Autodesk Inventor part; units mm, degrees
(part 4 of 4)
sketch "スケッチ30" plane through (0, 0, -5) normal (0, 0, -1) x (-1, 0, 0)
  arc A0 (-103.5253, -51.4545) -> (-102.2194, -50.4706) centre (-111.885, -39) ccw projected
  arc A1 (-103.5253, -51.4545) -> (-102.968, -53.2848) centre (-102.968, -52.2848) ccw projected
  line L0 (-102.968, -53.2848) -> (-61.8586, -53.2848) projected
  arc A2 (-61.8586, -53.2848) -> (-61.1613, -51.5681) centre (-61.8586, -52.2848) ccw projected
  line L1 (-61.1613, -51.5681) -> (-80.173, -33.0718) projected
  arc A3 (-80.173, -33.0718) -> (-81.5147, -33.0239) centre (-80.8703, -33.7886) ccw projected
  line L2 (-81.5147, -33.0239) -> (-102.2194, -50.4706) projected
  arc A4 (-99.1877, -14.5726) -> (-100.885, -15.2893) centre (-99.885, -15.2893) ccw projected
  line L3 (-100.885, -15.2893) -> (-100.885, -31.7889) projected
  arc A5 (-100.885, -31.7889) -> (-100.7422, -32.304) centre (-99.885, -31.7889) ccw projected
  arc A6 (-98.9442, -40.2383) -> (-100.7422, -32.304) centre (-111.885, -39) ccw projected
  arc A7 (-98.9442, -40.2383) -> (-97.3043, -41.0982) centre (-97.9487, -40.3335) ccw projected
  line L4 (-97.3043, -41.0982) -> (-84.5476, -30.3488) projected
  arc A8 (-84.5476, -30.3488) -> (-84.4946, -28.8673) centre (-85.1919, -29.5841) ccw projected
  line L5 (-84.4946, -28.8673) -> (-99.1877, -14.5726) projected
  arc A9 (-82.0469, -27.0631) -> (-80.7052, -27.1111) centre (-81.3496, -26.3464) ccw projected
  line L6 (-80.7052, -27.1111) -> (-61.3064, -10.7647) projected
  arc A10 (-61.3064, -10.7647) -> (-61.9507, -9) centre (-61.9507, -10) ccw projected
  line L7 (-61.9507, -9) -> (-62.4443, -9) projected
  arc A11 (-62.4443, -9) -> (-63.0443, -9.2) centre (-62.4443, -10) ccw projected
  arc A12 (-69.1163, -7.5865) -> (-63.0443, -9.2) centre (-65.4443, -6) ccw projected
  arc A13 (-69.1163, -7.5865) -> (-70.1163, -6.9865) centre (-70.0342, -7.9832) ccw projected
  arc A14 (-72.8443, -6.2) -> (-70.1163, -6.9865) centre (-70.4443, -3) ccw projected
  arc A15 (-72.8443, -6.2) -> (-73.4443, -6) centre (-73.4443, -7) ccw projected
  line L8 (-73.4443, -6) -> (-80.8897, -6) projected
  arc A16 (-80.8897, -6) -> (-81.4897, -6.2) centre (-80.8897, -7) ccw projected
  arc A17 (-84.2178, -6.9865) -> (-81.4897, -6.2) centre (-83.8897, -3) ccw projected
  arc A18 (-84.2178, -6.9865) -> (-85.2178, -7.5865) centre (-84.2998, -7.9832) ccw projected
  arc A19 (-91.2897, -9.2) -> (-85.2178, -7.5865) centre (-88.8897, -6) ccw projected
  arc A20 (-91.2897, -9.2) -> (-91.8897, -9) centre (-91.8897, -10) ccw projected
  line L9 (-91.8897, -9) -> (-92.8897, -9) projected
  arc A21 (-92.8897, -9) -> (-93.4897, -9.2) centre (-92.8897, -10) ccw projected
  arc A22 (-97.0553, -9.8264) -> (-93.4897, -9.2) centre (-95.8897, -6) ccw projected
  arc A23 (-97.0553, -9.8264) -> (-98.044, -11.4998) centre (-97.3467, -10.783) ccw projected
  line L10 (-98.044, -11.4998) -> (-82.0469, -27.0631) projected
  circle A24 centre (-90.0199, -69.8335) radius 1.5 projected
  circle A25 centre (-49.9722, -10.5) radius 1.5 projected
  arc A26 (-109.4606, -24.6009) -> (-107.885, -23.7831) centre (-108.885, -23.7831) ccw projected
  line L11 (-109.4606, -24.6009) -> (-113.2999, -21.8986) projected
  arc A27 (-113.5421, -20.5053) -> (-113.2999, -21.8986) centre (-112.7243, -21.0809) ccw projected
  line L12 (-113.5421, -20.5053) -> (-109.7028, -15.0506) projected
  arc A28 (-107.885, -15.6261) -> (-109.7028, -15.0506) centre (-108.885, -15.6261) ccw projected
  line L13 (-107.885, -15.6261) -> (-107.885, -23.7831) projected
  arc A29 (-118.0918, -32.7971) -> (-116.8906, -32.7594) centre (-117.5163, -31.9794) ccw projected
  line L14 (-118.0918, -32.7971) -> (-120.017, -31.4421) projected
  arc A30 (-120.2592, -30.0488) -> (-120.017, -31.4421) centre (-119.4414, -30.6244) ccw projected
  line L15 (-120.2592, -30.0488) -> (-116.4199, -24.5941) projected
  arc A31 (-115.0266, -24.3519) -> (-116.4199, -24.5941) centre (-115.6022, -25.1696) ccw projected
  line L16 (-115.0266, -24.3519) -> (-108.3095, -29.0797) projected
  arc A32 (-107.885, -29.8974) -> (-108.3095, -29.0797) centre (-108.885, -29.8974) ccw projected
  line L17 (-107.885, -29.8974) -> (-107.885, -30.5147) projected
  arc A33 (-109.2184, -31.4575) -> (-107.885, -30.5147) centre (-108.885, -30.5147) ccw projected
  arc A34 (-109.2184, -31.4575) -> (-116.8906, -32.7594) centre (-111.885, -39) ccw projected
  arc A35 (-121.5083, -34.0611) -> (-123.011, -34.5042) centre (-122.0839, -34.8788) ccw projected
  line L18 (-121.5083, -34.0611) -> (-119.8185, -35.2504) projected
  arc A36 (-119.4487, -36.3939) -> (-119.8185, -35.2504) centre (-120.3941, -36.0681) ccw projected
  arc A37 (-119.4487, -36.3939) -> (-119.4653, -41.5573) centre (-111.885, -39) ccw projected
  arc A38 (-120.4273, -42.8769) -> (-119.4653, -41.5573) centre (-120.4128, -41.877) ccw projected
  line L19 (-120.4273, -42.8769) -> (-123.2447, -42.8361) projected
  arc A39 (-124.2252, -41.735) -> (-123.2447, -42.8361) centre (-123.2303, -41.8362) ccw projected
  line L20 (-124.2252, -41.735) -> (-123.8235, -37.7857) projected
  arc A40 (-123.011, -34.5042) -> (-123.8235, -37.7857) centre (-111.885, -39) ccw projected
  arc A41 (-59.9987, -48.5136) -> (-58.3014, -47.7969) centre (-59.3014, -47.7969) ccw projected
  line L21 (-58.3014, -47.7969) -> (-58.3014, -15.6137) projected
  arc A42 (-58.3014, -15.6137) -> (-59.9457, -14.8489) centre (-59.3014, -15.6137) ccw projected
  line L22 (-59.9457, -14.8489) -> (-77.6723, -29.7862) projected
  arc A43 (-77.6723, -29.7862) -> (-77.7253, -31.2676) centre (-77.0279, -30.5509) ccw projected
  line L23 (-77.7253, -31.2676) -> (-59.9987, -48.5136) projected
  arc A44 (-65.1718, -84.4734) -> (-63.9261, -84.9061) centre (-64.3023, -83.9795) ccw projected
  line L24 (-63.9261, -84.9061) -> (-58.9251, -82.8752) projected
  arc A45 (-58.9251, -82.8752) -> (-58.3014, -81.9487) centre (-59.3014, -81.9487) ccw projected
  line L25 (-58.3014, -81.9487) -> (-58.3014, -57.2848) projected
  arc A46 (-58.3014, -57.2848) -> (-59.3014, -56.2848) centre (-59.3014, -57.2848) ccw projected
  line L26 (-59.3014, -56.2848) -> (-101.5991, -56.2848) projected
  arc A47 (-101.5991, -56.2848) -> (-102.1316, -58.1313) centre (-101.5991, -57.2848) ccw projected
  line L27 (-102.1316, -58.1313) -> (-90.9084, -65.1915) projected
  arc A48 (-90.9084, -65.1915) -> (-90.3112, -65.343) centre (-90.376, -64.3451) ccw projected
  arc A49 (-85.8458, -68.1521) -> (-90.3112, -65.343) centre (-90.0199, -69.8335) ccw projected
  arc A50 (-85.8458, -68.1521) -> (-85.4507, -68.6249) centre (-84.9182, -67.7784) ccw projected
  line L28 (-85.4507, -68.6249) -> (-72.5868, -76.7173) projected
  arc A51 (-65.1718, -84.4734) -> (-72.5868, -76.7173) centre (-84.3014, -95.339) ccw projected
  arc A52 (-62.421, -88.6121) -> (-63.0125, -89.7908) centre (-62.0448, -89.5386) ccw projected
  arc A53 (-62.7437, -90.9495) -> (-63.0125, -89.7908) centre (-84.3014, -95.339) ccw projected
  arc A54 (-62.7437, -90.9495) -> (-61.7638, -91.75) centre (-61.7638, -90.75) ccw projected
  line L29 (-61.7638, -91.75) -> (-55.2884, -91.75) projected
  arc A55 (-55.2884, -91.75) -> (-54.9084, -91.675) centre (-55.2884, -90.75) ccw projected
  line L30 (-54.9084, -91.675) -> (-53.6916, -91.1751) projected
  arc A56 (-53.6916, -91.1751) -> (-53.1201, -89.9424) centre (-54.0715, -90.2501) ccw projected
  arc A57 (-53.3763, -88.5912) -> (-53.1201, -89.9424) centre (-47.8869, -88.25) ccw projected
  arc A58 (-53.3763, -88.5912) -> (-54.1956, -87.6694) centre (-54.3744, -88.6533) ccw projected
  arc A59 (-56.3726, -86.6955) -> (-54.1956, -87.6694) centre (-53.3014, -82.75) ccw projected
  arc A60 (-56.3726, -86.6955) -> (-57.3632, -86.5581) centre (-56.9869, -87.4846) ccw projected
  line L31 (-57.3632, -86.5581) -> (-62.421, -88.6121) projected
  circle A61 centre (-47.8869, -88.25) radius 1.5 projected
  line L32 (-127.6513, -45.7727) -> (-119.127, -45.896) projected
  arc A62 (-119.127, -45.896) -> (-104.885, -31.8586) centre (-111.885, -39) ccw projected
  line L33 (-104.885, -31.8586) -> (-104.885, -3) projected
  line L34 (-104.885, -3) -> (-101.8897, -3) projected
  arc A63 (-101.8897, -3) -> (-99.8897, -3) centre (-100.8897, -3) ccw projected
  line L35 (-99.8897, -3) -> (-96.8897, -3) projected
  line L36 (-96.8897, -3) -> (-96.8897, -6) projected
  arc A64 (-96.8897, -6) -> (-94.8897, -6) centre (-95.8897, -6) ccw projected
  line L37 (-94.8897, -6) -> (-89.8897, -6) projected
  arc A65 (-89.8897, -6) -> (-87.8897, -6) centre (-88.8897, -6) ccw projected
  line L38 (-87.8897, -6) -> (-87.8897, -3) projected
  line L39 (-87.8897, -3) -> (-84.8897, -3) projected
  arc A66 (-84.8897, -3) -> (-82.8897, -3) centre (-83.8897, -3) ccw projected
  line L40 (-82.8897, -3) -> (-71.4443, -3) projected
  arc A67 (-71.4443, -3) -> (-69.4443, -3) centre (-70.4443, -3) ccw projected
  line L41 (-69.4443, -3) -> (-66.4443, -3) projected
  line L42 (-66.4443, -3) -> (-66.4443, -6) projected
  arc A68 (-66.4443, -6) -> (-64.4443, -6) centre (-65.4443, -6) ccw projected
  line L43 (-64.4443, -6) -> (-59.4443, -6) projected
  arc A69 (-59.4443, -6) -> (-57.4443, -6) centre (-58.4443, -6) ccw projected
  line L44 (-57.4443, -6) -> (-57.4443, -3) projected
  line L45 (-57.4443, -3) -> (-54.4443, -3) projected
  arc A70 (-54.4443, -3) -> (-52.4443, -3) centre (-53.4443, -3) ccw projected
  line L46 (-52.4443, -3) -> (-49.4443, -3) projected
  line L47 (-49.4443, -3) -> (-49.4443, -5.2165) projected
  arc A71 (-49.4443, -5.2165) -> (-48.7221, -6.1771) centre (-48.4443, -5.2165) ccw projected
  arc A72 (-52.6961, -14.082) -> (-48.7221, -6.1771) centre (-49.9722, -10.5) ccw projected
  arc A73 (-52.6961, -14.082) -> (-54.3014, -14.878) centre (-53.3014, -14.878) ccw projected
  line L48 (-54.3014, -14.878) -> (-54.3014, -82.75) projected
  arc A74 (-54.3014, -82.75) -> (-53.3014, -83.75) centre (-53.3014, -82.75) ccw projected
  line L49 (-53.3014, -83.75) -> (-47.885, -83.75) projected
  arc A75 (-46.177, -92.4125) -> (-47.885, -83.75) centre (-47.8869, -88.25) ccw projected
  line L50 (-46.177, -92.4125) -> (-54.3014, -95.75) projected
  line L51 (-54.3014, -95.75) -> (-66.3014, -95.75) projected
  line L52 (-66.3014, -95.75) -> (-66.3014, -95.339) projected
  arc A76 (-66.3014, -95.339) -> (-74.7167, -80.1031) centre (-84.3014, -95.339) ccw projected
  line L53 (-74.7167, -80.1031) -> (-85.8413, -73.1048) projected
  arc A77 (-85.8413, -73.1048) -> (-87.0367, -73.2026) centre (-86.3737, -73.9513) ccw projected
  arc A78 (-94.3483, -68.603) -> (-87.0367, -73.2026) centre (-90.0199, -69.8335) ccw projected
  arc A79 (-94.3483, -68.603) -> (-94.7777, -67.4831) centre (-95.3102, -68.3295) ccw projected
  line L54 (-94.7777, -67.4831) -> (-119.8722, -51.6966) projected
  arc A80 (-121.0577, -50.8686) -> (-119.8722, -51.6966) centre (-111.885, -39) ccw projected
  line L55 (-121.0577, -50.8686) -> (-127.6513, -45.7727) projected
  arc A81 (-52.6961, -14.082) -> (-54.3014, -14.878) centre (-53.3014, -14.878) ccw projected
  circle A82 centre (-49.9722, -10.5) radius 4.5
  line L56 (-54.3014, -14.878) -> (-54.3014, -9.2717)
  line L57 (-49.4443, -5.2165) -> (-49.4443, -3) projected
  line L58 (-49.4443, -5.2165) -> (-49.4443, -6.0311)
  point P0 (0, 0)
  constraints: 4 end point, 3 point on circle, 2 collinear, 1 centre point, 1 coincident
extrude "押し出し30" cut sketch "スケッチ30" against normal blind 2 contours L56 A82 A73 | A82 L56 A72 | A82 L58 A71
fillet "フィレット10" radius 1 1 edges at (54.3014, -9.2717, -4)
sketch "スケッチ31" plane through (0, 0, -5) normal (0, 0, -1) x (-1, 0, 0)
  arc A0 (-103.5253, -51.4545) -> (-102.2194, -50.4706) centre (-111.885, -39) ccw projected
  arc A1 (-103.5253, -51.4545) -> (-102.968, -53.2848) centre (-102.968, -52.2848) ccw projected
  line L0 (-102.968, -53.2848) -> (-61.8586, -53.2848) projected
  arc A2 (-61.8586, -53.2848) -> (-61.1613, -51.5681) centre (-61.8586, -52.2848) ccw projected
  line L1 (-61.1613, -51.5681) -> (-80.173, -33.0718) projected
  arc A3 (-80.173, -33.0718) -> (-81.5147, -33.0239) centre (-80.8703, -33.7886) ccw projected
  line L2 (-81.5147, -33.0239) -> (-102.2194, -50.4706) projected
  arc A4 (-99.1877, -14.5726) -> (-100.885, -15.2893) centre (-99.885, -15.2893) ccw projected
  line L3 (-100.885, -15.2893) -> (-100.885, -31.7889) projected
  arc A5 (-100.885, -31.7889) -> (-100.7422, -32.304) centre (-99.885, -31.7889) ccw projected
  arc A6 (-98.9442, -40.2383) -> (-100.7422, -32.304) centre (-111.885, -39) ccw projected
  arc A7 (-98.9442, -40.2383) -> (-97.3043, -41.0982) centre (-97.9487, -40.3335) ccw projected
  line L4 (-97.3043, -41.0982) -> (-84.5476, -30.3488) projected
  arc A8 (-84.5476, -30.3488) -> (-84.4946, -28.8673) centre (-85.1919, -29.5841) ccw projected
  line L5 (-84.4946, -28.8673) -> (-99.1877, -14.5726) projected
  arc A9 (-82.0469, -27.0631) -> (-80.7052, -27.1111) centre (-81.3496, -26.3464) ccw projected
  line L6 (-80.7052, -27.1111) -> (-61.3064, -10.7647) projected
  arc A10 (-61.3064, -10.7647) -> (-61.9507, -9) centre (-61.9507, -10) ccw projected
  line L7 (-61.9507, -9) -> (-62.4443, -9) projected
  arc A11 (-62.4443, -9) -> (-63.0443, -9.2) centre (-62.4443, -10) ccw projected
  arc A12 (-69.1163, -7.5865) -> (-63.0443, -9.2) centre (-65.4443, -6) ccw projected
  arc A13 (-69.1163, -7.5865) -> (-70.1163, -6.9865) centre (-70.0342, -7.9832) ccw projected
  arc A14 (-72.8443, -6.2) -> (-70.1163, -6.9865) centre (-70.4443, -3) ccw projected
  arc A15 (-72.8443, -6.2) -> (-73.4443, -6) centre (-73.4443, -7) ccw projected
  line L8 (-73.4443, -6) -> (-80.8897, -6) projected
  arc A16 (-80.8897, -6) -> (-81.4897, -6.2) centre (-80.8897, -7) ccw projected
  arc A17 (-84.2178, -6.9865) -> (-81.4897, -6.2) centre (-83.8897, -3) ccw projected
  arc A18 (-84.2178, -6.9865) -> (-85.2178, -7.5865) centre (-84.2998, -7.9832) ccw projected
  arc A19 (-91.2897, -9.2) -> (-85.2178, -7.5865) centre (-88.8897, -6) ccw projected
  arc A20 (-91.2897, -9.2) -> (-91.8897, -9) centre (-91.8897, -10) ccw projected
  line L9 (-91.8897, -9) -> (-92.8897, -9) projected
  arc A21 (-92.8897, -9) -> (-93.4897, -9.2) centre (-92.8897, -10) ccw projected
  arc A22 (-97.0553, -9.8264) -> (-93.4897, -9.2) centre (-95.8897, -6) ccw projected
  arc A23 (-97.0553, -9.8264) -> (-98.044, -11.4998) centre (-97.3467, -10.783) ccw projected
  line L10 (-98.044, -11.4998) -> (-82.0469, -27.0631) projected
  circle A24 centre (-90.0199, -69.8335) radius 1.5 projected
  arc A25 (-109.4606, -24.6009) -> (-107.885, -23.7831) centre (-108.885, -23.7831) ccw projected
  line L11 (-109.4606, -24.6009) -> (-113.2999, -21.8986) projected
  arc A26 (-113.5421, -20.5053) -> (-113.2999, -21.8986) centre (-112.7243, -21.0809) ccw projected
  line L12 (-113.5421, -20.5053) -> (-109.7028, -15.0506) projected
  arc A27 (-107.885, -15.6261) -> (-109.7028, -15.0506) centre (-108.885, -15.6261) ccw projected
  line L13 (-107.885, -15.6261) -> (-107.885, -23.7831) projected
  arc A28 (-118.0918, -32.7971) -> (-116.8906, -32.7594) centre (-117.5163, -31.9794) ccw projected
  line L14 (-118.0918, -32.7971) -> (-120.017, -31.4421) projected
  arc A29 (-120.2592, -30.0488) -> (-120.017, -31.4421) centre (-119.4414, -30.6244) ccw projected
  line L15 (-120.2592, -30.0488) -> (-116.4199, -24.5941) projected
  arc A30 (-115.0266, -24.3519) -> (-116.4199, -24.5941) centre (-115.6022, -25.1696) ccw projected
  line L16 (-115.0266, -24.3519) -> (-108.3095, -29.0797) projected
  arc A31 (-107.885, -29.8974) -> (-108.3095, -29.0797) centre (-108.885, -29.8974) ccw projected
  line L17 (-107.885, -29.8974) -> (-107.885, -30.5147) projected
  arc A32 (-109.2184, -31.4575) -> (-107.885, -30.5147) centre (-108.885, -30.5147) ccw projected
  arc A33 (-109.2184, -31.4575) -> (-116.8906, -32.7594) centre (-111.885, -39) ccw projected
  arc A34 (-121.5083, -34.0611) -> (-123.011, -34.5042) centre (-122.0839, -34.8788) ccw projected
  line L18 (-121.5083, -34.0611) -> (-119.8185, -35.2504) projected
  arc A35 (-119.4487, -36.3939) -> (-119.8185, -35.2504) centre (-120.3941, -36.0681) ccw projected
  arc A36 (-119.4487, -36.3939) -> (-119.4653, -41.5573) centre (-111.885, -39) ccw projected
  arc A37 (-120.4273, -42.8769) -> (-119.4653, -41.5573) centre (-120.4128, -41.877) ccw projected
  line L19 (-120.4273, -42.8769) -> (-123.2447, -42.8361) projected
  arc A38 (-124.2252, -41.735) -> (-123.2447, -42.8361) centre (-123.2303, -41.8362) ccw projected
  line L20 (-124.2252, -41.735) -> (-123.8235, -37.7857) projected
  arc A39 (-123.011, -34.5042) -> (-123.8235, -37.7857) centre (-111.885, -39) ccw projected
  arc A40 (-59.9987, -48.5136) -> (-58.3014, -47.7969) centre (-59.3014, -47.7969) ccw projected
  line L21 (-58.3014, -47.7969) -> (-58.3014, -15.6137) projected
  arc A41 (-58.3014, -15.6137) -> (-59.9457, -14.8489) centre (-59.3014, -15.6137) ccw projected
  line L22 (-59.9457, -14.8489) -> (-77.6723, -29.7862) projected
  arc A42 (-77.6723, -29.7862) -> (-77.7253, -31.2676) centre (-77.0279, -30.5509) ccw projected
  line L23 (-77.7253, -31.2676) -> (-59.9987, -48.5136) projected
  arc A43 (-65.1718, -84.4734) -> (-63.9261, -84.9061) centre (-64.3023, -83.9795) ccw projected
  line L24 (-63.9261, -84.9061) -> (-58.9251, -82.8752) projected
  arc A44 (-58.9251, -82.8752) -> (-58.3014, -81.9487) centre (-59.3014, -81.9487) ccw projected
  line L25 (-58.3014, -81.9487) -> (-58.3014, -57.2848) projected
  arc A45 (-58.3014, -57.2848) -> (-59.3014, -56.2848) centre (-59.3014, -57.2848) ccw projected
  line L26 (-59.3014, -56.2848) -> (-101.5991, -56.2848) projected
  arc A46 (-101.5991, -56.2848) -> (-102.1316, -58.1313) centre (-101.5991, -57.2848) ccw projected
  line L27 (-102.1316, -58.1313) -> (-90.9084, -65.1915) projected
  arc A47 (-90.9084, -65.1915) -> (-90.3112, -65.343) centre (-90.376, -64.3451) ccw projected
  arc A48 (-85.8458, -68.1521) -> (-90.3112, -65.343) centre (-90.0199, -69.8335) ccw projected
  arc A49 (-85.8458, -68.1521) -> (-85.4507, -68.6249) centre (-84.9182, -67.7784) ccw projected
  line L28 (-85.4507, -68.6249) -> (-72.5868, -76.7173) projected
  arc A50 (-65.1718, -84.4734) -> (-72.5868, -76.7173) centre (-84.3014, -95.339) ccw projected
  arc A51 (-62.421, -88.6121) -> (-63.0125, -89.7908) centre (-62.0448, -89.5386) ccw projected
  arc A52 (-62.7437, -90.9495) -> (-63.0125, -89.7908) centre (-84.3014, -95.339) ccw projected
  arc A53 (-62.7437, -90.9495) -> (-61.7638, -91.75) centre (-61.7638, -90.75) ccw projected
  line L29 (-61.7638, -91.75) -> (-55.2884, -91.75) projected
  arc A54 (-55.2884, -91.75) -> (-54.9084, -91.675) centre (-55.2884, -90.75) ccw projected
  line L30 (-54.9084, -91.675) -> (-53.6916, -91.1751) projected
  arc A55 (-53.6916, -91.1751) -> (-53.1201, -89.9424) centre (-54.0715, -90.2501) ccw projected
  arc A56 (-53.3763, -88.5912) -> (-53.1201, -89.9424) centre (-47.8869, -88.25) ccw projected
  arc A57 (-53.3763, -88.5912) -> (-54.1956, -87.6694) centre (-54.3744, -88.6533) ccw projected
  arc A58 (-56.3726, -86.6955) -> (-54.1956, -87.6694) centre (-53.3014, -82.75) ccw projected
  arc A59 (-56.3726, -86.6955) -> (-57.3632, -86.5581) centre (-56.9869, -87.4846) ccw projected
  line L31 (-57.3632, -86.5581) -> (-62.421, -88.6121) projected
  circle A60 centre (-47.8869, -88.25) radius 1.5 projected
  line L32 (-127.6513, -45.7727) -> (-119.127, -45.896) projected
  arc A61 (-119.127, -45.896) -> (-104.885, -31.8586) centre (-111.885, -39) ccw projected
  line L33 (-104.885, -31.8586) -> (-104.885, -3) projected
  line L34 (-104.885, -3) -> (-101.8897, -3) projected
  arc A62 (-101.8897, -3) -> (-99.8897, -3) centre (-100.8897, -3) ccw projected
  line L35 (-99.8897, -3) -> (-96.8897, -3) projected
  line L36 (-96.8897, -3) -> (-96.8897, -6) projected
  arc A63 (-96.8897, -6) -> (-94.8897, -6) centre (-95.8897, -6) ccw projected
  line L37 (-94.8897, -6) -> (-89.8897, -6) projected
  arc A64 (-89.8897, -6) -> (-87.8897, -6) centre (-88.8897, -6) ccw projected
  line L38 (-87.8897, -6) -> (-87.8897, -3) projected
  line L39 (-87.8897, -3) -> (-84.8897, -3) projected
  arc A65 (-84.8897, -3) -> (-82.8897, -3) centre (-83.8897, -3) ccw projected
  line L40 (-82.8897, -3) -> (-71.4443, -3) projected
  arc A66 (-71.4443, -3) -> (-69.4443, -3) centre (-70.4443, -3) ccw projected
  line L41 (-69.4443, -3) -> (-66.4443, -3) projected
  line L42 (-66.4443, -3) -> (-66.4443, -6) projected
  arc A67 (-66.4443, -6) -> (-64.4443, -6) centre (-65.4443, -6) ccw projected
  line L43 (-64.4443, -6) -> (-59.4443, -6) projected
  arc A68 (-59.4443, -6) -> (-57.4443, -6) centre (-58.4443, -6) ccw projected
  line L44 (-57.4443, -6) -> (-57.4443, -3) projected
  line L45 (-57.4443, -3) -> (-54.4443, -3) projected
  arc A69 (-54.4443, -3) -> (-52.4443, -3) centre (-53.4443, -3) ccw projected
  line L46 (-52.4443, -3) -> (-49.4443, -3) projected
  line L47 (-49.4443, -3) -> (-49.4443, -6.0311) projected
  arc A70 (-49.4443, -6.0311) -> (-54.2525, -9.111) centre (-49.9722, -10.5) ccw projected
  arc A71 (-54.2525, -9.111) -> (-54.3014, -9.4197) centre (-53.3014, -9.4197) ccw projected
  line L48 (-54.3014, -9.4197) -> (-54.3014, -82.75) projected
  arc A72 (-54.3014, -82.75) -> (-53.3014, -83.75) centre (-53.3014, -82.75) ccw projected
  line L49 (-53.3014, -83.75) -> (-47.885, -83.75) projected
  arc A73 (-46.177, -92.4125) -> (-47.885, -83.75) centre (-47.8869, -88.25) ccw projected
  line L50 (-46.177, -92.4125) -> (-54.3014, -95.75) projected
  line L51 (-54.3014, -95.75) -> (-66.3014, -95.75) projected
  line L52 (-66.3014, -95.75) -> (-66.3014, -95.339) projected
  arc A74 (-66.3014, -95.339) -> (-74.7167, -80.1031) centre (-84.3014, -95.339) ccw projected
  line L53 (-74.7167, -80.1031) -> (-85.8413, -73.1048) projected
  arc A75 (-85.8413, -73.1048) -> (-87.0367, -73.2026) centre (-86.3737, -73.9513) ccw projected
  arc A76 (-94.3483, -68.603) -> (-87.0367, -73.2026) centre (-90.0199, -69.8335) ccw projected
  arc A77 (-94.3483, -68.603) -> (-94.7777, -67.4831) centre (-95.3102, -68.3295) ccw projected
  line L54 (-94.7777, -67.4831) -> (-119.8722, -51.6966) projected
  arc A78 (-121.0577, -50.8686) -> (-119.8722, -51.6966) centre (-111.885, -39) ccw projected
  line L55 (-121.0577, -50.8686) -> (-127.6513, -45.7727) projected
  line L56 (-54.4443, 0.873) -> (-54.4443, -6)
  arc A79 (-61.3905, -8.7056) -> (-54.4443, -6) centre (-58.4443, -6) ccw
  arc A80 (-68.5345, -6) -> (-63.1683, -8.0901) centre (-65.4443, -6) ccw
  line L57 (-68.5345, -6) -> (-68.5345, -0.5707)
  arc A81 (-72.7204, -5.0901) -> (-68.5345, -0.5707) centre (-70.4443, -3) ccw
  line L58 (-72.7204, -5.0901) -> (-81.6137, -5.0901)
  arc A82 (-85.7996, -0.5707) -> (-81.6137, -5.0901) centre (-83.8897, -3) ccw
  line L59 (-85.7996, -0.5707) -> (-85.7996, -6)
  arc A83 (-91.1657, -8.0901) -> (-85.7996, -6) centre (-88.8897, -6) ccw
  line L60 (-91.1657, -8.0901) -> (-93.6137, -8.0901)
  arc A84 (-98.9798, -6) -> (-93.6137, -8.0901) centre (-95.8897, -6) ccw
  line L61 (-98.9798, -6) -> (-98.9798, -0.5707)
  arc A85 (-102.7949, -0.5671) -> (-98.9798, -0.5707) centre (-100.8897, -3) ccw
  line L62 (-102.7949, -0.5671) -> (-102.7949, -31.0288)
  arc A86 (-119.9869, -47.9739) -> (-102.7949, -31.0288) centre (-111.885, -39) ccw
  line L63 (-119.9869, -47.9739) -> (-121.4118, -47.9533)
  line L64 (-121.4118, -47.9533) -> (-119.7795, -49.2148)
  arc A87 (-119.7795, -49.2148) -> (-118.7593, -49.9275) centre (-111.885, -39) ccw
  line L65 (-118.7593, -49.9275) -> (-93.6648, -65.7139)
  arc A88 (-92.3379, -69.1745) -> (-93.6648, -65.7139) centre (-95.3102, -68.3295) ccw
  arc A89 (-92.3379, -69.1745) -> (-88.4223, -71.6378) centre (-90.0199, -69.8335) ccw
  arc A90 (-84.7283, -71.3357) -> (-88.4223, -71.6378) centre (-86.3737, -73.9513) ccw
  line L66 (-84.7283, -71.3357) -> (-73.6038, -78.3339)
  arc A91 (-64.2815, -93.6599) -> (-73.6038, -78.3339) centre (-84.3014, -95.339) ccw
  line L67 (-64.2815, -93.6599) -> (-54.7139, -93.6599)
  line L68 (-54.7139, -93.6599) -> (-46.9712, -90.4791)
  arc A92 (-46.9712, -90.4791) -> (-47.8869, -85.8401) centre (-47.8869, -88.25) ccw
  line L69 (-47.8869, -85.8401) -> (-53.3014, -85.8401)
  arc A93 (-56.3915, -82.75) -> (-53.3014, -85.8401) centre (-53.3014, -82.75) ccw
  arc A94 (-57.1061, -8.1851) -> (-57.3014, -9.4197) centre (-53.3014, -9.4197) ccw
  arc A95 (-43.9722, -6) -> (-57.1061, -8.1851) centre (-49.9722, -10.5) ccw
  line L70 (-43.9722, -6) -> (-50.7986, -6)
  arc A96 (-54.4443, 0.873) -> (-50.7986, -6) centre (-53.4443, -3) ccw
  line L71 (-54.3014, -82.75) -> (-54.3014, -9.4197) projected
  line L72 (-54.3014, -9.4197) -> (-54.3014, -5.4047)
  point P0 (0, 0)
  point P1 (-52.7158, -6.9331)
  point P2 (-54.3014, -6.9071)
  dimension "d221" = 3
  dimension "d222" = 3
  constraints: 36 point on circle, 32 end point, 18 centre point, 1 collinear, 30 other
  measures "d221" radial gap between concentric circles of A69 A96
  measures "d222" distance between parallel lines of L44 L56
extrude "押し出し31" cut sketch "スケッチ31" against normal blind 2 contours L72 A96 A70 A71
fillet "フィレット11" radius 1 1 edges at (54.3014, -6.9071, -4)
sketch "スケッチ32" plane through (0, 0, 0) normal (0, 0, 1) x (1, 0, 0)
  arc A0 (54.3014, -7.998) -> (53.33, -6.9984) centre (53.3014, -7.998) ccw projected
  line L0 (54.3014, -14.878) -> (54.3014, -7.998) projected
  arc A1 (54.3014, -14.878) -> (52.6961, -14.082) centre (53.3014, -14.878) ccw projected
  arc A2 (48.7221, -6.1771) -> (52.6961, -14.082) centre (49.9722, -10.5) ccw projected
  arc A3 (48.7221, -6.1771) -> (49.4443, -5.2165) centre (48.4443, -5.2165) ccw projected
  line L1 (49.4443, -6.0311) -> (49.4443, -5.2165) projected
  arc A4 (52.7158, -6.9331) -> (49.4443, -6.0311) centre (49.9722, -10.5) ccw projected
  arc A5 (52.7158, -6.9331) -> (53.33, -6.9984) centre (53.4443, -3) ccw projected
  circle A6 centre (49.9722, -10.5) radius 1.5 projected
  point P0 (0, 0)
sketch "スケッチ33" plane through (0, 0, -3) normal (0, 0, -1) x (-1, 0, 0)
  arc A0 (-103.5253, -51.4545) -> (-102.2194, -50.4706) centre (-111.885, -39) ccw projected
  arc A1 (-103.5253, -51.4545) -> (-102.968, -53.2848) centre (-102.968, -52.2848) ccw projected
  line L0 (-102.968, -53.2848) -> (-61.8586, -53.2848) projected
  arc A2 (-61.8586, -53.2848) -> (-61.1613, -51.5681) centre (-61.8586, -52.2848) ccw projected
  line L1 (-61.1613, -51.5681) -> (-80.173, -33.0718) projected
  arc A3 (-80.173, -33.0718) -> (-81.5147, -33.0239) centre (-80.8703, -33.7886) ccw projected
  line L2 (-81.5147, -33.0239) -> (-102.2194, -50.4706) projected
  arc A4 (-99.1877, -14.5726) -> (-100.885, -15.2893) centre (-99.885, -15.2893) ccw projected
  line L3 (-100.885, -15.2893) -> (-100.885, -31.7889) projected
  arc A5 (-100.885, -31.7889) -> (-100.7422, -32.304) centre (-99.885, -31.7889) ccw projected
  arc A6 (-98.9442, -40.2383) -> (-100.7422, -32.304) centre (-111.885, -39) ccw projected
  arc A7 (-98.9442, -40.2383) -> (-97.3043, -41.0982) centre (-97.9487, -40.3335) ccw projected
  line L4 (-97.3043, -41.0982) -> (-84.5476, -30.3488) projected
  arc A8 (-84.5476, -30.3488) -> (-84.4946, -28.8673) centre (-85.1919, -29.5841) ccw projected
  line L5 (-84.4946, -28.8673) -> (-99.1877, -14.5726) projected
  arc A9 (-82.0469, -27.0631) -> (-80.7052, -27.1111) centre (-81.3496, -26.3464) ccw projected
  line L6 (-80.7052, -27.1111) -> (-61.3064, -10.7647) projected
  arc A10 (-61.3064, -10.7647) -> (-61.9507, -9) centre (-61.9507, -10) ccw projected
  line L7 (-61.9507, -9) -> (-62.4443, -9) projected
  arc A11 (-62.4443, -9) -> (-63.0443, -9.2) centre (-62.4443, -10) ccw projected
  arc A12 (-69.1163, -7.5865) -> (-63.0443, -9.2) centre (-65.4443, -6) ccw projected
  arc A13 (-69.1163, -7.5865) -> (-70.1163, -6.9865) centre (-70.0342, -7.9832) ccw projected
  arc A14 (-72.8443, -6.2) -> (-70.1163, -6.9865) centre (-70.4443, -3) ccw projected
  arc A15 (-72.8443, -6.2) -> (-73.4443, -6) centre (-73.4443, -7) ccw projected
  line L8 (-73.4443, -6) -> (-80.8897, -6) projected
  arc A16 (-80.8897, -6) -> (-81.4897, -6.2) centre (-80.8897, -7) ccw projected
  arc A17 (-84.2178, -6.9865) -> (-81.4897, -6.2) centre (-83.8897, -3) ccw projected
  arc A18 (-84.2178, -6.9865) -> (-85.2178, -7.5865) centre (-84.2998, -7.9832) ccw projected
  arc A19 (-91.2897, -9.2) -> (-85.2178, -7.5865) centre (-88.8897, -6) ccw projected
  arc A20 (-91.2897, -9.2) -> (-91.8897, -9) centre (-91.8897, -10) ccw projected
  line L9 (-91.8897, -9) -> (-92.8897, -9) projected
  arc A21 (-92.8897, -9) -> (-93.4897, -9.2) centre (-92.8897, -10) ccw projected
  arc A22 (-97.0553, -9.8264) -> (-93.4897, -9.2) centre (-95.8897, -6) ccw projected
  arc A23 (-97.0553, -9.8264) -> (-98.044, -11.4998) centre (-97.3467, -10.783) ccw projected
  line L10 (-98.044, -11.4998) -> (-82.0469, -27.0631) projected
  circle A24 centre (-90.0199, -69.8335) radius 1.5 projected
  circle A25 centre (-49.9722, -10.5) radius 1.5 projected
  arc A26 (-109.4606, -24.6009) -> (-107.885, -23.7831) centre (-108.885, -23.7831) ccw projected
  line L11 (-109.4606, -24.6009) -> (-113.2999, -21.8986) projected
  arc A27 (-113.5421, -20.5053) -> (-113.2999, -21.8986) centre (-112.7243, -21.0809) ccw projected
  line L12 (-113.5421, -20.5053) -> (-109.7028, -15.0506) projected
  arc A28 (-107.885, -15.6261) -> (-109.7028, -15.0506) centre (-108.885, -15.6261) ccw projected
  line L13 (-107.885, -15.6261) -> (-107.885, -23.7831) projected
  arc A29 (-118.0918, -32.7971) -> (-116.8906, -32.7594) centre (-117.5163, -31.9794) ccw projected
  line L14 (-118.0918, -32.7971) -> (-120.017, -31.4421) projected
  arc A30 (-120.2592, -30.0488) -> (-120.017, -31.4421) centre (-119.4414, -30.6244) ccw projected
  line L15 (-120.2592, -30.0488) -> (-116.4199, -24.5941) projected
  arc A31 (-115.0266, -24.3519) -> (-116.4199, -24.5941) centre (-115.6022, -25.1696) ccw projected
  line L16 (-115.0266, -24.3519) -> (-108.3095, -29.0797) projected
  arc A32 (-107.885, -29.8974) -> (-108.3095, -29.0797) centre (-108.885, -29.8974) ccw projected
  line L17 (-107.885, -29.8974) -> (-107.885, -30.5147) projected
  arc A33 (-109.2184, -31.4575) -> (-107.885, -30.5147) centre (-108.885, -30.5147) ccw projected
  arc A34 (-109.2184, -31.4575) -> (-116.8906, -32.7594) centre (-111.885, -39) ccw projected
  arc A35 (-121.5083, -34.0611) -> (-123.011, -34.5042) centre (-122.0839, -34.8788) ccw projected
  line L18 (-121.5083, -34.0611) -> (-119.8185, -35.2504) projected
  arc A36 (-119.4487, -36.3939) -> (-119.8185, -35.2504) centre (-120.3941, -36.0681) ccw projected
  arc A37 (-119.4487, -36.3939) -> (-119.4653, -41.5573) centre (-111.885, -39) ccw projected
  arc A38 (-120.4273, -42.8769) -> (-119.4653, -41.5573) centre (-120.4128, -41.877) ccw projected
  line L19 (-120.4273, -42.8769) -> (-123.2447, -42.8361) projected
  arc A39 (-124.2252, -41.735) -> (-123.2447, -42.8361) centre (-123.2303, -41.8362) ccw projected
  line L20 (-124.2252, -41.735) -> (-123.8235, -37.7857) projected
  arc A40 (-123.011, -34.5042) -> (-123.8235, -37.7857) centre (-111.885, -39) ccw projected
  arc A41 (-59.9987, -48.5136) -> (-58.3014, -47.7969) centre (-59.3014, -47.7969) ccw projected
  line L21 (-58.3014, -47.7969) -> (-58.3014, -15.6137) projected
  arc A42 (-58.3014, -15.6137) -> (-59.9457, -14.8489) centre (-59.3014, -15.6137) ccw projected
  line L22 (-59.9457, -14.8489) -> (-77.6723, -29.7862) projected
  arc A43 (-77.6723, -29.7862) -> (-77.7253, -31.2676) centre (-77.0279, -30.5509) ccw projected
  line L23 (-77.7253, -31.2676) -> (-59.9987, -48.5136) projected
  arc A44 (-65.1718, -84.4734) -> (-63.9261, -84.9061) centre (-64.3023, -83.9795) ccw projected
  line L24 (-63.9261, -84.9061) -> (-58.9251, -82.8752) projected
  arc A45 (-58.9251, -82.8752) -> (-58.3014, -81.9487) centre (-59.3014, -81.9487) ccw projected
  line L25 (-58.3014, -81.9487) -> (-58.3014, -57.2848) projected
  arc A46 (-58.3014, -57.2848) -> (-59.3014, -56.2848) centre (-59.3014, -57.2848) ccw projected
  line L26 (-59.3014, -56.2848) -> (-101.5991, -56.2848) projected
  arc A47 (-101.5991, -56.2848) -> (-102.1316, -58.1313) centre (-101.5991, -57.2848) ccw projected
  line L27 (-102.1316, -58.1313) -> (-90.9084, -65.1915) projected
  arc A48 (-90.9084, -65.1915) -> (-90.3112, -65.343) centre (-90.376, -64.3451) ccw projected
  arc A49 (-85.8458, -68.1521) -> (-90.3112, -65.343) centre (-90.0199, -69.8335) ccw projected
  arc A50 (-85.8458, -68.1521) -> (-85.4507, -68.6249) centre (-84.9182, -67.7784) ccw projected
  line L28 (-85.4507, -68.6249) -> (-72.5868, -76.7173) projected
  arc A51 (-65.1718, -84.4734) -> (-72.5868, -76.7173) centre (-84.3014, -95.339) ccw projected
  arc A52 (-62.421, -88.6121) -> (-63.0125, -89.7908) centre (-62.0448, -89.5386) ccw projected
  arc A53 (-62.7437, -90.9495) -> (-63.0125, -89.7908) centre (-84.3014, -95.339) ccw projected
  arc A54 (-62.7437, -90.9495) -> (-61.7638, -91.75) centre (-61.7638, -90.75) ccw projected
  line L29 (-61.7638, -91.75) -> (-55.2884, -91.75) projected
  arc A55 (-55.2884, -91.75) -> (-54.9084, -91.675) centre (-55.2884, -90.75) ccw projected
  line L30 (-54.9084, -91.675) -> (-53.6916, -91.1751) projected
  arc A56 (-53.6916, -91.1751) -> (-53.1201, -89.9424) centre (-54.0715, -90.2501) ccw projected
  arc A57 (-53.3763, -88.5912) -> (-53.1201, -89.9424) centre (-47.8869, -88.25) ccw projected
  arc A58 (-53.3763, -88.5912) -> (-54.1956, -87.6694) centre (-54.3744, -88.6533) ccw projected
  arc A59 (-56.3726, -86.6955) -> (-54.1956, -87.6694) centre (-53.3014, -82.75) ccw projected
  arc A60 (-56.3726, -86.6955) -> (-57.3632, -86.5581) centre (-56.9869, -87.4846) ccw projected
  line L31 (-57.3632, -86.5581) -> (-62.421, -88.6121) projected
  circle A61 centre (-47.8869, -88.25) radius 1.5 projected
  line L32 (-127.6513, -45.7727) -> (-119.127, -45.896) projected
  arc A62 (-119.127, -45.896) -> (-104.885, -31.8586) centre (-111.885, -39) ccw projected
  line L33 (-104.885, -31.8586) -> (-104.885, -3) projected
  line L34 (-104.885, -3) -> (-101.8897, -3) projected
  arc A63 (-101.8897, -3) -> (-99.8897, -3) centre (-100.8897, -3) ccw projected
  line L35 (-99.8897, -3) -> (-96.8897, -3) projected
  arc A64 (-94.8897, -3) -> (-96.8897, -3) centre (-95.8897, -3) ccw projected
  line L36 (-89.8897, -3) -> (-94.8897, -3) projected
  arc A65 (-87.8897, -3) -> (-89.8897, -3) centre (-88.8897, -3) ccw projected
  line L37 (-87.8897, -6) -> (-87.8897, -3) projected
  arc A66 (-89.8897, -6) -> (-87.8897, -6) centre (-88.8897, -6) ccw projected
  line L38 (-94.8897, -6) -> (-89.8897, -6) projected
  arc A67 (-96.8897, -6) -> (-94.8897, -6) centre (-95.8897, -6) ccw projected
  line L39 (-96.8897, -3) -> (-96.8897, -6) projected
  line L40 (-121.0577, -50.8686) -> (-127.6513, -45.7727) projected
  arc A68 (-121.0577, -50.8686) -> (-119.8722, -51.6966) centre (-111.885, -39) ccw projected
  line L41 (-94.7777, -67.4831) -> (-119.8722, -51.6966) projected
  arc A69 (-94.3483, -68.603) -> (-94.7777, -67.4831) centre (-95.3102, -68.3295) ccw projected
  arc A70 (-94.3483, -68.603) -> (-87.0367, -73.2026) centre (-90.0199, -69.8335) ccw projected
  arc A71 (-85.8413, -73.1048) -> (-87.0367, -73.2026) centre (-86.3737, -73.9513) ccw projected
  line L42 (-74.7167, -80.1031) -> (-85.8413, -73.1048) projected
  arc A72 (-66.3014, -95.339) -> (-74.7167, -80.1031) centre (-84.3014, -95.339) ccw projected
  line L43 (-66.3014, -95.75) -> (-66.3014, -95.339) projected
  line L44 (-54.3014, -95.75) -> (-66.3014, -95.75) projected
  line L45 (-46.177, -92.4125) -> (-54.3014, -95.75) projected
  arc A73 (-46.177, -92.4125) -> (-47.885, -83.75) centre (-47.8869, -88.25) ccw projected
  line L46 (-53.3014, -83.75) -> (-47.885, -83.75) projected
  arc A74 (-54.3014, -82.75) -> (-53.3014, -83.75) centre (-53.3014, -82.75) ccw projected
  line L47 (-54.3014, -14.878) -> (-54.3014, -82.75) projected
  arc A75 (-52.6961, -14.082) -> (-54.3014, -14.878) centre (-53.3014, -14.878) ccw projected
  arc A76 (-52.6961, -14.082) -> (-48.7221, -6.1771) centre (-49.9722, -10.5) ccw projected
  arc A77 (-49.4443, -5.2165) -> (-48.7221, -6.1771) centre (-48.4443, -5.2165) ccw projected
  line L48 (-49.4443, -5.2165) -> (-49.4443, -6.0311) projected
  arc A78 (-49.4443, -6.0311) -> (-52.7158, -6.9331) centre (-49.9722, -10.5) ccw projected
  arc A79 (-53.33, -6.9984) -> (-52.7158, -6.9331) centre (-53.4443, -3) ccw projected
  arc A80 (-53.33, -6.9984) -> (-54.3014, -7.998) centre (-53.3014, -7.998) ccw projected
  line L49 (-54.3014, -7.998) -> (-54.3014, -14.878) projected
  line L50 (-99.8897, -3) -> (-99.8897, 0) projected
  line L51 (-99.8897, 0) -> (-84.8897, 0) projected
  line L52 (-84.8897, 0) -> (-84.8897, -3) projected
  line L53 (-87.8897, -3) -> (-84.8897, -3) projected
  line L54 (-49.4443, -3) -> (-49.4443, -5.2165) projected
  line L55 (-52.4443, -3) -> (-49.4443, -3) projected
  arc A81 (-54.4443, -3) -> (-52.4443, -3) centre (-53.4443, -3) ccw projected
  line L56 (-54.4443, 0) -> (-54.4443, -3) projected
  line L57 (-69.4443, 0) -> (-54.4443, 0) projected
  line L58 (-69.4443, -3) -> (-69.4443, 0) projected
  line L59 (-69.4443, -3) -> (-66.4443, -3) projected
  line L60 (-66.4443, -3) -> (-66.4443, -6) projected
  arc A82 (-66.4443, -6) -> (-64.4443, -6) centre (-65.4443, -6) ccw projected
  line L61 (-64.4443, -6) -> (-59.4443, -6) projected
  arc A83 (-59.4443, -6) -> (-57.4443, -6) centre (-58.4443, -6) ccw projected
  line L62 (-57.4443, -6) -> (-57.4443, -3) projected
  line L63 (-57.4443, -3) -> (-54.4443, -3) projected
  arc A84 (-84.8897, -3) -> (-82.8897, -3) centre (-83.8897, -3) ccw projected
  line L64 (-82.8897, -3) -> (-71.4443, -3) projected
  arc A85 (-71.4443, -3) -> (-69.4443, -3) centre (-70.4443, -3) ccw projected
  arc A86 (-64.4443, -3) -> (-66.4443, -3) centre (-65.4443, -3) ccw projected
  line L65 (-59.4443, -3) -> (-64.4443, -3) projected
  arc A87 (-57.4443, -3) -> (-59.4443, -3) centre (-58.4443, -3) ccw projected
  circle A88 centre (-49.9722, -10.5) radius 3
  point P0 (0, 0)
  dimension "d226" = 6
  constraints: 1 centre point, 1 coincident
  measures "d226" diameter of A88
extrude "押し出し32" cut sketch "スケッチ33" against normal blind 0.4 contours A88
equation "\"d9\" = d7"
equation "\"d26\" = d7"
